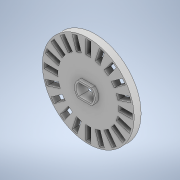
# Autodesk Inventor part: ХЗ контроллер там блин
Saved by Autodesk Inventor 2021 (Build 250183000, 183)
## iProperties
Created: 2022-07-09
Part Number: ХЗ контроллер там блин
Material: Типовые
Document SubType Name: Modeling
Designer: zvi20
Density: 1 g/cm^3
Appearance: По умолчанию
Author: zvi20
Autodesk Inventor part; units mm, degrees
ref_plane "YZ Plane" through (0, 0, 0) normal (1, 0, 0) x (0, 1, 0)
ref_plane "XZ Plane" through (0, 0, 0) normal (0, 1, 0) x (-1, 0, 0)
ref_plane "XY Plane" through (0, 0, 0) normal (0, 0, 1) x (1, 0, 0)
sketch "Эскиз1" plane through (0, 0, 0) normal (0, 0, 1) x (1, 0, 0)
  circle A0 centre (25.264, -13.4877) radius 13.25
  line L0 (25.264, -11.7377) -> (27.0494, -11.7377)
  line L1 (27.0494, -11.7377) -> (23.4787, -11.7377)
  line L2 (25.264, -15.2377) -> (23.4787, -15.2377)
  line L3 (23.4787, -15.2377) -> (27.0494, -15.2377)
  arc A1 (23.4787, -11.7377) -> (23.4787, -15.2377) centre (25.264, -13.4877) ccw
  arc A2 (27.0494, -15.2377) -> (27.0494, -11.7377) centre (25.264, -13.4877) ccw
  line L4 (25.264, -11.2377) -> (27.2484, -11.2377)
  line L5 (23.2797, -11.2377) -> (27.2484, -11.2377)
  line L6 (25.264, -15.7377) -> (27.2484, -15.7377)
  line L7 (27.2484, -15.7377) -> (23.2797, -15.7377)
  arc A3 (27.2484, -15.7377) -> (27.2484, -11.2377) centre (25.264, -13.4877) ccw
  arc A4 (23.2797, -11.2377) -> (23.2797, -15.7377) centre (25.264, -13.4877) ccw
  line L8 (25.264, -0.7377) -> (26.014, -0.7377)
  line L9 (26.014, -0.7377) -> (24.514, -0.7377)
  line L10 (24.514, -0.7377) -> (24.514, -4.7377)
  line L11 (24.514, -4.7377) -> (26.014, -4.7377)
  line L12 (26.014, -4.7377) -> (26.014, -0.7377)
  line L13 (21.8469, -5.3978) -> (23.2734, -4.9342)
  line L14 (23.2734, -4.9342) -> (22.0374, -1.13)
  line L15 (21.3241, -1.3618) -> (22.0374, -1.13)
  line L16 (22.0374, -1.13) -> (20.6108, -1.5935)
  line L17 (20.6108, -1.5935) -> (21.8469, -5.3978)
  line L18 (19.5142, -6.8497) -> (20.7277, -5.968)
  line L19 (20.7277, -5.968) -> (18.3765, -2.7319)
  line L20 (17.7698, -3.1728) -> (18.3765, -2.7319)
  line L21 (18.3765, -2.7319) -> (17.163, -3.6136)
  line L22 (17.163, -3.6136) -> (19.5142, -6.8497)
  line L23 (17.7443, -8.9514) -> (18.626, -7.7379)
  line L24 (18.626, -7.7379) -> (15.3899, -5.3867)
  line L25 (14.9491, -5.9935) -> (15.3899, -5.3867)
  line L26 (15.3899, -5.3867) -> (14.5082, -6.6002)
  line L27 (14.5082, -6.6002) -> (17.7443, -8.9514)
  line L28 (16.7105, -11.4971) -> (17.1741, -10.0705)
  line L29 (17.1741, -10.0705) -> (13.3698, -8.8345)
  line L30 (13.1381, -9.5478) -> (13.3698, -8.8345)
  line L31 (13.3698, -8.8345) -> (12.9063, -10.2611)
  line L32 (12.9063, -10.2611) -> (16.7105, -11.4971)
  line L33 (16.514, -14.2377) -> (16.514, -12.7377)
  line L34 (16.514, -12.7377) -> (12.514, -12.7377)
  line L35 (12.514, -13.4877) -> (12.514, -12.7377)
  line L36 (12.514, -12.7377) -> (12.514, -14.2377)
  line L37 (12.514, -14.2377) -> (16.514, -14.2377)
  line L38 (17.1741, -16.9049) -> (16.7105, -15.4783)
  line L39 (16.7105, -15.4783) -> (12.9063, -16.7144)
  line L40 (13.1381, -17.4277) -> (12.9063, -16.7144)
  line L41 (12.9063, -16.7144) -> (13.3698, -18.141)
  line L42 (13.3698, -18.141) -> (17.1741, -16.9049)
  line L43 (18.626, -19.2376) -> (17.7443, -18.0241)
  line L44 (17.7443, -18.0241) -> (14.5082, -20.3752)
  line L45 (14.9491, -20.982) -> (14.5082, -20.3752)
  line L46 (14.5082, -20.3752) -> (15.3899, -21.5888)
  line L47 (15.3899, -21.5888) -> (18.626, -19.2376)
  line L48 (20.7277, -21.0075) -> (19.5142, -20.1258)
  line L49 (19.5142, -20.1258) -> (17.163, -23.3619)
  line L50 (17.7698, -23.8027) -> (17.163, -23.3619)
  line L51 (17.163, -23.3619) -> (18.3765, -24.2435)
  line L52 (18.3765, -24.2435) -> (20.7277, -21.0075)
  line L53 (23.2734, -22.0412) -> (21.8469, -21.5777)
  line L54 (21.8469, -21.5777) -> (20.6108, -25.3819)
  line L55 (21.3241, -25.6137) -> (20.6108, -25.3819)
  line L56 (20.6108, -25.3819) -> (22.0374, -25.8455)
  line L57 (22.0374, -25.8455) -> (23.2734, -22.0412)
  line L58 (26.014, -22.2377) -> (24.514, -22.2377)
  line L59 (24.514, -22.2377) -> (24.514, -26.2377)
  line L60 (25.264, -26.2377) -> (24.514, -26.2377)
  line L61 (24.514, -26.2377) -> (26.014, -26.2377)
  line L62 (26.014, -26.2377) -> (26.014, -22.2377)
  line L63 (28.6812, -21.5777) -> (27.2546, -22.0412)
  line L64 (27.2546, -22.0412) -> (28.4907, -25.8455)
  line L65 (29.204, -25.6137) -> (28.4907, -25.8455)
  line L66 (28.4907, -25.8455) -> (29.9173, -25.3819)
  line L67 (29.9173, -25.3819) -> (28.6812, -21.5777)
  line L68 (31.0139, -20.1258) -> (29.8004, -21.0075)
  line L69 (29.8004, -21.0075) -> (32.1515, -24.2435)
  line L70 (32.7583, -23.8027) -> (32.1515, -24.2435)
  line L71 (32.1515, -24.2435) -> (33.3651, -23.3619)
  line L72 (33.3651, -23.3619) -> (31.0139, -20.1258)
  line L73 (32.7838, -18.0241) -> (31.9021, -19.2376)
  line L74 (31.9021, -19.2376) -> (35.1382, -21.5888)
  line L75 (35.579, -20.982) -> (35.1382, -21.5888)
  line L76 (35.1382, -21.5888) -> (36.0198, -20.3752)
  line L77 (36.0198, -20.3752) -> (32.7838, -18.0241)
  line L78 (33.8175, -15.4783) -> (33.354, -16.9049)
  line L79 (33.354, -16.9049) -> (37.1582, -18.141)
  line L80 (37.39, -17.4277) -> (37.1582, -18.141)
  line L81 (37.1582, -18.141) -> (37.6218, -16.7144)
  line L82 (37.6218, -16.7144) -> (33.8175, -15.4783)
  line L83 (34.014, -12.7377) -> (34.014, -14.2377)
  line L84 (34.014, -14.2377) -> (38.014, -14.2377)
  line L85 (38.014, -13.4877) -> (38.014, -14.2377)
  line L86 (38.014, -14.2377) -> (38.014, -12.7377)
  line L87 (38.014, -12.7377) -> (34.014, -12.7377)
  line L88 (33.354, -10.0705) -> (33.8175, -11.4971)
  line L89 (33.8175, -11.4971) -> (37.6218, -10.2611)
  line L90 (37.39, -9.5478) -> (37.6218, -10.2611)
  line L91 (37.6218, -10.2611) -> (37.1582, -8.8345)
  line L92 (37.1582, -8.8345) -> (33.354, -10.0705)
  line L93 (31.9021, -7.7379) -> (32.7838, -8.9514)
  line L94 (32.7838, -8.9514) -> (36.0198, -6.6002)
  line L95 (35.579, -5.9935) -> (36.0198, -6.6002)
  line L96 (36.0198, -6.6002) -> (35.1382, -5.3867)
  line L97 (35.1382, -5.3867) -> (31.9021, -7.7379)
  line L98 (29.8004, -5.968) -> (31.0139, -6.8497)
  line L99 (31.0139, -6.8497) -> (33.3651, -3.6136)
  line L100 (32.7583, -3.1728) -> (33.3651, -3.6136)
  line L101 (33.3651, -3.6136) -> (32.1515, -2.7319)
  line L102 (32.1515, -2.7319) -> (29.8004, -5.968)
  line L103 (27.2546, -4.9342) -> (28.6812, -5.3978)
  line L104 (28.6812, -5.3978) -> (29.9173, -1.5935)
  line L105 (29.204, -1.3618) -> (29.9173, -1.5935)
  line L106 (29.9173, -1.5935) -> (28.4907, -1.13)
  line L107 (28.4907, -1.13) -> (27.2546, -4.9342)
  point P0 (0, 0)
  dimension "d9" = 0.75
  dimension "d10" = 1.5
  dimension "d11" = 4
  dimension "d12" = 1.5
  dimension "d15" = 360
  constraints: 216 end point, 23 point on line, 8 point on circle, 5 centre point, 2 coincident, 2 perpendicular, 1 collinear, 1 horizontal, 201 other
  measures "d9" distance of L8.start L8.end
  measures "d10" distance of L8.end L9.end
  measures "d11" distance of L9.end L10.end
  measures "d12" distance of L10.end L11.end
extrude "Выдавливание1" add sketch "Эскиз1" along normal blind 2 contours A0
extrude "Выдавливание2" add sketch "Эскиз1" along normal blind 3 contours L4 A3 L6 L7 A4 L5
